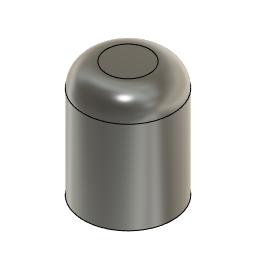
Button v2 (Autodesk Fusion 360 design; units mm, degrees)
Autodesk Fusion 360 part; units mm, degrees
cylinder "CylinderPrimitive1" add diameter 7.7 height 5 placed x (1, 0, 0) y (0, 1, 0) z (0, 0, 1) at (0, 0, 0)
extrude "Extrude1" add 1 faces at (-0.2155, 0.3161, 5) along direction (0, 0, 1) blind 5
fillet "Fillet1" radius 2 1 edges at (-3.5895, -1.3922, 10)
